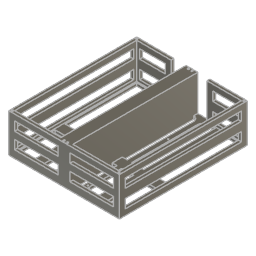
Boite Batterie (Autodesk Fusion 360 design; units mm, degrees)
Autodesk Fusion 360 part; units mm, degrees
sketch "Esquisse1" plane through (0, 0, 0) normal (0, 0, 1) x (1, 0, 0)
  line L0 (0, 0) -> (83, 0)
  line L1 (83, 0) -> (83, 205)
  line L2 (83, 205) -> (0, 205)
  line L3 (0, 205) -> (0, 0)
  line L4 (0, 205) -> (-5, 205)
  line L5 (83, 205) -> (82, 205)
  line L6 (-5, 205) -> (88, 205)
  line L7 (88, 205) -> (88, 210)
  line L8 (88, 210) -> (-5, 210)
  line L9 (-5, 210) -> (-5, 205)
  line L10 (88, -5) -> (-5, -5)
  line L11 (-5, 205) -> (-5, -5)
  line L12 (88, 205) -> (88, -5)
  dimension "d1" = 83
  dimension "d2" = 205
  dimension "d74" = 5
  dimension "d75" = 5
  dimension "d76" = 5
  dimension "d77" = 5
  constraint horizontal L0
  constraint vertical L1
  constraint horizontal L2
  constraint vertical L3
  constraint horizontal L4
  constraint horizontal L5
  constraint horizontal L6
  constraint vertical L7
  constraint horizontal L8
  constraint vertical L9
  constraint horizontal L10
  constraint perpendicular L4 L11
  constraint perpendicular L10 L12
  constraint coincident L0.start L3.end
  measures "d1" distance of L1.end L2.end
  measures "d2" distance of L0.end L1.end
  measures "d74" distance of L3 L11
  measures "d75" distance of L6 L8
  measures "d76" distance of L1 L12
  measures "d77" distance of L0 L10
extrude "Extrusion1" add sketch "Esquisse1" along normal blind 65 contours L0 L1 L3 L4 L6 L10 L11 L12 | L2 L4 L5 L6 L7 L8 L9
extrude "Extrusion2" add sketch "Esquisse1" along normal blind 5 contours L0 L1 L2 L3 L5 L6
sketch "Esquisse3" plane through (0, 210, 0) normal (0, 1, 0) x (-1, 0, 0)
  line L0 (-88, 0) -> (5, 0)
  line L1 (5, 0) -> (5, 65)
  line L2 (5, 65) -> (-88, 65)
  line L3 (-88, 65) -> (-88, 0)
  line L4 (-25, 65) -> (-5, 65)
  line L5 (-5, 65) -> (-5, 0)
  line L6 (-5, 0) -> (-25, 0)
  line L7 (-25, 0) -> (-25, 65)
  line L8 (-25, 5) -> (-5, 5)
  dimension "d13" = 10
  dimension "d14" = 20
  dimension "d17" = 5
  constraint horizontal L4
  constraint vertical L5
  constraint horizontal L6
  constraint vertical L7
  constraint coincident L0 L5.end
  constraint coincident L2 L4.start
  constraint coincident L7 L8.start
  constraint coincident L5 L8.end
  constraint perpendicular L5 L8
  measures "d13" distance of L1 L5
  measures "d14" distance of L4.start L4.end
  measures "d17" distance of L6 L8
extrude "Extrusion3" cut sketch "Esquisse3" against normal blind 40 contours L2 L4 L5 L7 L8
sketch "Esquisse5" plane through (88, 0, 0) normal (1, 0, 0) x (0, 1, 0)
  line L0 (-5, 0) -> (210, 0)
  line L1 (210, 65) -> (-5, 65)
  line L2 (-5, 65) -> (-5, 0)
  line L3 (-5, 65) -> (210, 65)
  line L4 (210, 65) -> (210, 0)
  line L5 (210, 0) -> (-5, 0)
  line L6 (-5, 0) -> (-5, 65)
  line L7 (5, 55) -> (200, 55)
  line L8 (200, 55) -> (200, 40)
  line L9 (200, 40) -> (5, 40)
  line L10 (5, 40) -> (5, 55)
  line L11 (5, 25) -> (200, 25)
  line L12 (200, 25) -> (200, 10)
  line L13 (200, 10) -> (5, 10)
  line L14 (5, 10) -> (5, 25)
  dimension "d181" = 15
  dimension "d182" = 15
  dimension "d183" = 10
  dimension "d185" = 10
  dimension "d186" = 10
  dimension "d187" = 10
  dimension "d188" = 10
  dimension "d189" = 10
  constraint horizontal L3
  constraint vertical L4
  constraint horizontal L5
  constraint vertical L6
  constraint coincident L0.end L4.end
  constraint coincident L1.end L2.start
  constraint horizontal L7
  constraint vertical L8
  constraint horizontal L9
  constraint vertical L10
  constraint horizontal L11
  constraint vertical L12
  constraint horizontal L13
  constraint vertical L14
  measures "d181" distance of L7 L9
  measures "d182" distance of L11 L13
  measures "d183" distance of L3 L7
  measures "d185" distance of L6 L10
  measures "d186" distance of L4 L8
  measures "d187" distance of L4 L12
  measures "d188" distance of L6 L14
  measures "d189" distance of L5 L13
extrude "Extrusion5" cut sketch "Esquisse5" against normal blind 155 contours L7 L8 L9 L10 | L11 L12 L13 L14
sketch "Esquisse6" plane through (0, -5, 0) normal (0, -1, 0) x (1, 0, 0)
  line L0 (-5, 0) -> (88, 0)
  line L1 (88, 0) -> (88, 65)
  line L2 (88, 65) -> (-5, 65)
  line L3 (-5, 65) -> (-5, 0)
  line L4 (-5, 65) -> (88, 65)
  line L5 (88, 65) -> (88, 0)
  line L6 (88, 0) -> (-5, 0)
  line L7 (-5, 0) -> (-5, 65)
  line L8 (5, 55) -> (78, 55)
  line L9 (78, 55) -> (78, 40)
  line L10 (78, 40) -> (5, 40)
  line L11 (5, 40) -> (5, 55)
  line L12 (5, 28) -> (78, 28)
  line L13 (78, 28) -> (78, 13)
  line L14 (78, 13) -> (5, 13)
  line L15 (5, 13) -> (5, 28)
  dimension "d199" = 10
  dimension "d200" = 12
  dimension "d201" = 15
  dimension "d202" = 15
  dimension "d203" = 10
  dimension "d204" = 10
  dimension "d205" = 10
  dimension "d206" = 10
  constraint horizontal L4
  constraint vertical L5
  constraint horizontal L6
  constraint vertical L7
  constraint coincident L0.end L1.start
  constraint coincident L2.end L3.start
  constraint horizontal L8
  constraint vertical L9
  constraint horizontal L10
  constraint vertical L11
  constraint horizontal L12
  constraint vertical L13
  constraint horizontal L14
  constraint vertical L15
  measures "d199" distance of L4 L8
  measures "d200" distance of L10 L12
  measures "d201" distance of L8.end L9.end
  measures "d202" distance of L12.end L13.end
  measures "d203" distance of L7 L11
  measures "d204" distance of L5 L9
  measures "d205" distance of L5 L13
  measures "d206" distance of L7 L15
extrude "Extrusion6" cut sketch "Esquisse6" against normal blind 20 contours L8 L9 L10 L11 | L12 L13 L14 L15
sketch "Esquisse7" plane through (0, 210, 0) normal (0, 1, 0) x (-1, 0, 0)
  line L0 (-25, 5) -> (-25, 65)
  line L1 (-88, 0) -> (5, 0)
  line L2 (5, 0) -> (5, 65)
  line L3 (5, 65) -> (-5, 65)
  line L4 (-5, 65) -> (-5, 5)
  line L5 (-5, 5) -> (-25, 5)
  line L6 (-13, 32.5, -10) -> (-13, 32.5, 0)
  line L7 (-25, 65) -> (-88, 65)
  line L8 (-88, 65) -> (-88, 0)
  line L9 (-88, 0) -> (-25, 0)
  line L10 (-25, 0) -> (-25, 65)
  line L11 (-78, 55) -> (-35, 55)
  line L12 (-35, 55) -> (-35, 40)
  line L13 (-35, 40) -> (-78, 40)
  line L14 (-78, 40) -> (-78, 55)
  line L15 (-78, 25) -> (-35, 25)
  line L16 (-35, 25) -> (-35, 10)
  line L17 (-35, 10) -> (-78, 10)
  line L18 (-78, 10) -> (-78, 25)
  point P0 (-13, 32.5)
  dimension "d207" = 10
  dimension "d208" = 10
  dimension "d209" = 15
  dimension "d210" = 15
  dimension "d211" = 10
  dimension "d212" = 10
  dimension "d213" = 10
  dimension "d214" = 10
  constraint horizontal L7
  constraint vertical L8
  constraint horizontal L9
  constraint vertical L10
  constraint coincident L1.start L8.end
  constraint coincident L0.end L7.start
  constraint horizontal L11
  constraint vertical L12
  constraint horizontal L13
  constraint vertical L14
  constraint horizontal L15
  constraint vertical L16
  constraint horizontal L17
  constraint vertical L18
  measures "d207" distance of L7 L11
  measures "d208" distance of L9 L17
  measures "d209" distance of L13 L15
  measures "d210" distance of L11.end L12.end
  measures "d211" distance of L10 L12
  measures "d212" distance of L8 L14
  measures "d213" distance of L10 L16
  measures "d214" distance of L8 L18
extrude "Extrusion7" cut sketch "Esquisse7" against normal blind 50 contours L11 L12 L13 L14 | L15 L16 L17 L18
sketch "Esquisse8" plane through (0, 0, 0) normal (0, 0, -1) x (1, 0, 0)
  line L0 (88, 5) -> (-5, 5)
  line L1 (-5, -210) -> (88, -210)
  line L2 (88, -210) -> (88, 5)
  line L3 (88, 5) -> (-5, 5)
  line L4 (-5, 5) -> (-5, -210)
  line L5 (5, -2) -> (81, -2)
  line L6 (81, -2) -> (81, -203)
  line L7 (81, -203) -> (5, -203)
  line L8 (5, -203) -> (5, -2)
  line L9 (13, -2) -> (21, -2)
  line L10 (21, -2) -> (21, -203)
  line L11 (21, -203) -> (13, -203)
  line L12 (13, -203) -> (13, -2)
  line L13 (31, -2) -> (41, -2)
  line L14 (41, -2) -> (41, -203)
  line L15 (41, -203) -> (31, -203)
  line L16 (31, -203) -> (31, -2)
  line L17 (56, -2) -> (66, -2)
  line L18 (66, -2) -> (66, -203)
  line L19 (66, -203) -> (56, -203)
  line L20 (56, -203) -> (56, -2)
  dimension "d99" = 10
  dimension "d100" = 7
  dimension "d101" = 7
  dimension "d102" = 7
  dimension "d103" = 8
  dimension "d104" = 10
  dimension "d105" = 10
  dimension "d106" = 15
  dimension "d107" = 10
  dimension "d108" = 8
  constraint horizontal L5
  constraint vertical L6
  constraint horizontal L7
  constraint vertical L8
  constraint horizontal L9
  constraint vertical L10
  constraint horizontal L11
  constraint vertical L12
  constraint coincident L7 L10.end
  constraint coincident L5 L9.start
  constraint horizontal L13
  constraint vertical L14
  constraint horizontal L15
  constraint vertical L16
  constraint coincident L7 L14.end
  constraint coincident L5 L13.start
  constraint horizontal L17
  constraint vertical L18
  constraint horizontal L19
  constraint vertical L20
  constraint coincident L7 L18.end
  constraint coincident L5 L17.start
  measures "d99" distance of L4 L8
  measures "d100" distance of L2 L6
  measures "d101" distance of L0 L5
  measures "d102" distance of L1 L7
  measures "d103" distance of L9.start L9.end
  measures "d104" distance of L9.end L13.start
  measures "d105" distance of L13.start L13.end
  measures "d106" distance of L13.end L17.start
  measures "d107" distance of L17.start L17.end
  measures "d108" distance of L8 L12
extrude "Extrusion8" cut sketch "Esquisse8" against normal blind 25 contours L5 L7 L8 L12 | L5 L7 L10 L16 | L5 L7 L13 L14 L15 L16 | L5 L7 L17 L18 L19 L20 | L5 L6 L7 L18
sketch "Esquisse9" plane through (0, 0, 0) normal (0, 0, -1) x (1, 0, 0)
  line L0 (-5, -210) -> (88, -210)
  line L1 (88, -210) -> (88, 5)
  line L2 (88, 5) -> (-5, 5)
  line L3 (-5, 5) -> (-5, -210)
  circle A0 centre (17.5, -12.5) radius 1
  circle A1 centre (17.5, -147.5) radius 1
  circle A2 centre (50, -62.5) radius 1
  circle A3 centre (50, -87.5) radius 1
  line L4 (21, -203) -> (21, -2)
  line L5 (41, -203) -> (21, -203)
  line L6 (41, -2) -> (41, -203)
  line L7 (21, -2) -> (41, -2)
  line L8 (56, -203) -> (56, -2)
  line L9 (13, -2) -> (13, -203)
  line L10 (13, -203) -> (5, -203)
  line L11 (5, -203) -> (5, -2)
  line L12 (5, -2) -> (13, -2)
  line L13 (81, -2) -> (81, -203)
  line L14 (81, -203) -> (56, -203)
  line L15 (56, -2) -> (81, -2)
  dimension "d60" = 2
  dimension "d61" = 22.5
  dimension "d62" = 17.5
  dimension "d63" = 2
  dimension "d64" = 22.5
  dimension "d65" = 135
  dimension "d68" = 2
  dimension "d69" = 55
  dimension "d70" = 50
  dimension "d71" = 2
  dimension "d72" = 25
  dimension "d73" = 55
  measures "d60" diameter of A0
  measures "d61" distance of L3 A0.centre
  measures "d62" distance of L2 A0.centre
  measures "d63" diameter of A1
  measures "d64" distance of L3 A1.centre
  measures "d65" distance of A0.centre A1.centre
  measures "d68" diameter of A2
  measures "d69" distance of L3 A2.centre
  measures "d70" vertical distance of A0.centre A2.centre
  measures "d71" diameter of A3
  measures "d72" vertical distance of A2.centre A3.centre
  measures "d73" distance of L3 A3.centre
extrude "Extrusion9" cut sketch "Esquisse9" against normal blind 10 contours A0 | A1 | A2 | A3
fillet "Congé1" radius 10 1 edges at (21, 2, 2.5)
fillet "Congé2" radius 8 1 edges at (13, 2, 2.5)
fillet "Congé3" radius 8 1 edges at (13, 203, 2.5)
fillet "Congé4" radius 10 1 edges at (21, 203, 2.5)
ref_plane "Plan de construction1" through (-5, 102.5, 32.5) normal (-1, 0, 0) x (0, -1, 0)
sketch "Esquisse11" plane through (0, 0, 65) normal (0, 0, 1) x (-1, 0, 0)
  line L0 (-83, -205) -> (-83, 0)
  line L1 (-83, 0) -> (0, 0)
  line L2 (0, 0) -> (0, -205)
  line L3 (-5, -205) -> (-5, -210)
  line L4 (-5, -210) -> (5, -210)
  line L5 (5, 5) -> (-88, 5)
  line L6 (-88, 5) -> (-88, -210)
  line L7 (0, -210) -> (-5, -210)
  line L8 (-5, -210) -> (-5, 5)
  line L9 (-5, 5) -> (0, 5)
  line L10 (0, 5) -> (0, -210)
  line L11 (-25, -205) -> (-83, -205)
  line L12 (5, -210) -> (5, 5)
  line L13 (-25, -210) -> (-25, -205)
  line L14 (0, -205) -> (-5, -205)
  line L15 (-88, -210) -> (-25, -210)
  dimension "d126" = 5
  dimension "d127" = 5
  constraint horizontal L7
  constraint vertical L8
  constraint horizontal L9
  constraint vertical L10
  constraint coincident L5 L8.end
  constraint coincident L4 L7.start
  measures "d126" distance of L7.start L3.end
  measures "d127" distance of L4.end L7.start
extrude "Extrusion10" add sketch "Esquisse11" against normal blind 60 contours L1 L5 L8 L9 L10 | L1 L2 L8 L10 L14 | L3 L4 L7 L8 L10 L14
sketch "Esquisse12" plane through (0, 0, 65) normal (0, 0, 1) x (-1, 0, 0)
  line L0 (-88, -210) -> (-25, -210)
  line L1 (-83, 0) -> (-5, 0)
  line L2 (-5, 0) -> (-5, -210)
  line L3 (-87.8203, -207) -> (-87.8203, -207.0054)
  line L4 (-87.8203, -207) -> (-88, -207)
  line L5 (5, 5) -> (-88, 5)
  line L6 (-88, 5) -> (-88, -210)
  line L7 (5, -210) -> (5, 5)
  line L8 (-88, -210) -> (-25, -210)
  line L9 (-5, -210) -> (5, -210)
  line L10 (5, -210) -> (-88, -210)
  line L11 (-88, -210) -> (-88, 5)
  line L12 (-88, 5) -> (5, 5)
  line L13 (5, 5) -> (5, -210)
  line L14 (-88, 5) -> (-85, 5)
  line L15 (-85, 5) -> (-85, 2)
  line L16 (-85, 2) -> (-88, 2)
  line L17 (-88, 2) -> (-88, 5)
  circle A0 centre (-85, 2) radius 1.5
  line L18 (-88, -210) -> (-85, -210)
  line L19 (-85, -210) -> (-85, -207)
  line L20 (-85, -207) -> (-88, -207)
  line L21 (-88, -207) -> (-88, -210)
  circle A1 centre (-85, -207) radius 1.5
  line L22 (5, -210) -> (2, -210)
  line L23 (2, -210) -> (2, -207)
  line L24 (2, -207) -> (5, -207)
  line L25 (5, -207) -> (5, -210)
  circle A2 centre (2, -207) radius 1.5
  line L26 (5, 5) -> (2, 5)
  line L27 (2, 5) -> (2, 2)
  line L28 (2, 2) -> (5, 2)
  line L29 (5, 2) -> (5, 5)
  circle A3 centre (2, 2) radius 1.5
  point P0 (-87.8203, -207)
  point P1 (-56.5, -210)
  dimension "d215" = 3
  dimension "d216" = 3
  dimension "d217" = 3
  dimension "d218" = 3
  dimension "d219" = 3
  dimension "d220" = 3
  dimension "d221" = 3
  dimension "d222" = 3
  dimension "d223" = 3
  dimension "d224" = 3
  dimension "d225" = 3
  dimension "d226" = 3
  constraint coincident P0 L3.start
  constraint midpoint L0 P1
  constraint horizontal L10
  constraint vertical L11
  constraint horizontal L12
  constraint vertical L13
  constraint coincident L5.end L6.start
  constraint coincident L7.start L9.end
  constraint horizontal L14
  constraint vertical L15
  constraint horizontal L16
  constraint vertical L17
  constraint coincident L15.end L16.start
  constraint horizontal L18
  constraint vertical L19
  constraint horizontal L20
  constraint vertical L21
  constraint coincident L0.start L6.end
  constraint coincident L19.end L20.start
  constraint horizontal L22
  constraint vertical L23
  constraint horizontal L24
  constraint vertical L25
  constraint coincident L23.end L24.start
  constraint horizontal L26
  constraint vertical L27
  constraint horizontal L28
  constraint vertical L29
  constraint coincident L5.start L7.end
  constraint coincident L27.end L28.start
  measures "d215" distance of L5.end L14.end
  measures "d216" distance of L5.end L16.end
  measures "d217" diameter of A0
  measures "d218" distance of L0.start L18.end
  measures "d219" distance of L0.start L4.end
  measures "d220" diameter of A1
  measures "d221" distance of L23.end L24.end
  measures "d222" distance of L7.start L24.end
  measures "d223" diameter of A2
  measures "d224" distance of L5.start L28.end
  measures "d225" distance of L5.start L26.end
  measures "d226" diameter of A3
extrude "Extrusion11" cut sketch "Esquisse12" against normal blind 8 contours L19 L20 A1 | L19 L20 A1 | L15 L16 A0 | L15 L16 A0 | L23 L24 A2 | L23 L24 A2 | L27 L28 A3 | L27 L28 A3
mirror "Symétrie miroir2" about plane through (-5, 102.5, 32.5) normal (-1, 0, 0) of bodies 1 merged
sketch "Esquisse13" plane through (0, 0, 0) normal (0, 0, -1) x (1, 0, 0)
  arc A0 (-23, -195) -> (-15, -203) centre (-15, -195) ccw
  line L0 (-23, -195) -> (-23, -10)
  arc A1 (-15, -2) -> (-23, -10) centre (-15, -10) ccw
  circle A2 centre (-27.5, -147.5) radius 1
  circle A3 centre (-60, -62.5) radius 1
  circle A4 centre (-27.5, -12.5) radius 1
  circle A5 centre (-60, -87.5) radius 1
  line L1 (-41, -203) -> (-51, -203)
  line L2 (-51, -203) -> (-51, -2)
  line L3 (-51, -2) -> (-41, -2)
  arc A6 (-31, -12) -> (-41, -2) centre (-41, -12) ccw
  line L4 (-31, -12) -> (-31, -193)
  arc A7 (-41, -203) -> (-31, -193) centre (-41, -193) ccw
  line L5 (-91, -203) -> (-91, -2)
  line L6 (-91, -2) -> (-66, -2)
  line L7 (-66, -2) -> (-66, -203)
  line L8 (-66, -203) -> (-91, -203)
  line L9 (-98, -210) -> (88, -210)
  line L10 (88, -210) -> (88, 5)
  line L11 (88, 5) -> (-98, 5)
  line L12 (-98, 5) -> (-98, -210)
  line L13 (81, -2) -> (81, -203)
  line L14 (81, -203) -> (56, -203)
  line L15 (56, -203) -> (56, -2)
  line L16 (56, -2) -> (81, -2)
  line L17 (41, -203) -> (31, -203)
  arc A8 (21, -193) -> (31, -203) centre (31, -193) ccw
  line L18 (21, -193) -> (21, -12)
  arc A9 (31, -2) -> (21, -12) centre (31, -12) ccw
  line L19 (31, -2) -> (41, -2)
  line L20 (41, -2) -> (41, -203)
  circle A10 centre (50, -87.5) radius 1
  circle A11 centre (17.5, -12.5) radius 1
  circle A12 centre (50, -62.5) radius 1
  circle A13 centre (17.5, -147.5) radius 1
  arc A14 (13, -10) -> (5, -2) centre (5, -10) ccw
  line L21 (13, -10) -> (13, -195)
  arc A15 (5, -203) -> (13, -195) centre (5, -195) ccw
  line L22 (-91, -66) -> (88, -66)
  line L23 (-91, -83) -> (88, -83)
  line L24 (-91, -66) -> (-98, -66)
  line L25 (-91, -83) -> (-98, -83)
  line L26 (-15, -2) -> (-15, -203)
  line L27 (5, -203) -> (5, -2)
  dimension "d177" = 17
  dimension "d178" = 71
  constraint coincident L5 L22.start
  constraint coincident L10 L22.end
  constraint perpendicular L10 L22
  constraint coincident L5 L23.start
  constraint coincident L10 L23.end
  constraint perpendicular L10 L23
  constraint coincident L12 L24.end
  constraint perpendicular L12 L24
  constraint coincident L12 L25.end
  constraint perpendicular L12 L25
  measures "d177" distance of L22.start L23.start
  measures "d178" distance of L11 L22
extrude "Extrusion12" add sketch "Esquisse13" against normal blind 5 contours L0 L4 L22 L23 | L0 L22 L23 L26 | L22 L23 L26 L27 | L2 L4 L22 L23 | L21 L22 L23 L27 | L2 L7 L22 L23 | L18 L21 L22 L23 | L5 L7 L22 L23 | L18 L20 L22 L23 | L5 L12 L24 L25 | L15 L20 L22 L23 | L13 L15 L22 L23 | L10 L13 L22 L23
